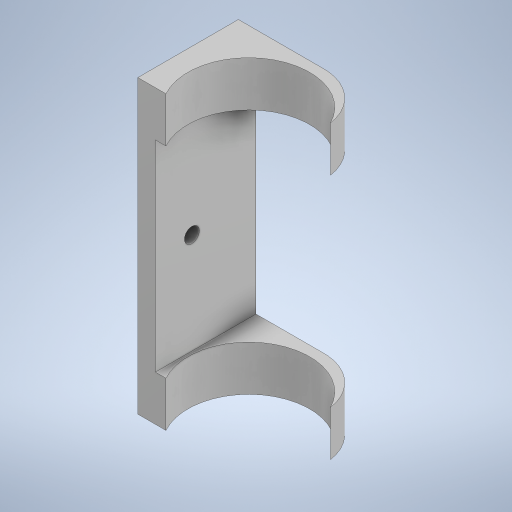
# Autodesk Inventor part: Speed Champ
Saved by Autodesk Inventor 2024 (Build 280153000, 153)
## iProperties
Created: 2023-08-06
Part Number: Speed Champ
Material: Generic
Document SubType Name: Modeling
Designer: AdminForWorker
Density: 1 g/cm^3
Appearance: Default
Title: Speed Champ v1
Author: AdminForWorker
Autodesk Inventor part; units mm, degrees
ref_plane "YZ Plane" through (0, 0, 0) normal (1, 0, 0) x (0, 1, 0)
ref_plane "Work Plane1" through (-14.5, -35, 0) normal (0, -1, 0) x (1, 0, 0)
sketch "Sketch2" plane through (-14.5, -35, 0) normal (0, -1, 0) x (1, 0, 0)
  line L0 (4.3469, 0) -> (4.3469, 20)
  line L1 (7.596, 20) -> (7.4184, 20) projected
  line L2 (4.3469, 20) -> (7.596, 20)
  arc A0 (7.596, 20) -> (29, 8.6937) centre (18.17, 14.1045) ccw
  line L3 (4.3469, 0) -> (18.3998, 0)
  arc A1 (18.3998, 0) -> (29, 8.6937) centre (18.9461, 10.1431) ccw
  point P0 (14.5, 0)
  point P1 (5, 0)
  point P2 (18.2531, 1.9984)
  constraints: 6 end point, 5 point on circle, 2 centre point, 1 horizontal, 1 perpendicular
extrude "Extrusion1" add sketch "Sketch2" against normal blind 15
ref_plane "Work Plane4" through (-14.5, -35, 0) normal (-1, 0, 0) x (0, 0, 1)
sketch "Sketch3" plane through (-14.5, -35, 0) normal (-1, 0, 0) x (0, 0, 1)
  line L0 (20, 0) -> (20, 70) projected
  line L1 (0, 0) -> (0, 21) projected
  line L2 (20, 70) -> (0, 70)
  line L3 (0, 70) -> (0, 0)
  line L4 (0, 0) -> (20, 0)
  line L5 (20, 0) -> (20, 70)
  point P0 (0, 35)
  constraints: 8 end point, 2 parallel, 1 horizontal, 1 perpendicular
extrude "Extrusion2" add sketch "Sketch3" against normal blind 5.5
mirror "Mirror3" about plane through (0, 0, 0) normal (0, 1, 0) of "Extrusion1"
sketch "Sketch4" plane through (-9, -35, 0) normal (1, 0, 0) x (0, 0, -1)
  line L0 (-20, 15) -> (-1.9981, 15) projected
  line L1 (-12.7438, 15) -> (-12.7438, 55)
  line L2 (0, 55) -> (-20, 55) projected
  line L3 (-12.7438, 35) -> (-17.7089, 35)
  circle A0 centre (-12.7438, 35) radius 1.5
  point P0 (0, 35)
  point P1 (-8.6937, 15)
  dimension "d4" = 3
  constraints: 4 end point, 2 point on line, 1 centre point, 1 coincident, 1 horizontal, 1 midpoint, 1 vertical
  measures "d4" diameter of A0
extrude "Extrusion3" cut sketch "Sketch4" against normal blind 10.375
sketch "Sketch5" plane through (-14.5, -35, 0) normal (-1, 0, 0) x (0, 0, 1)
  line L0 (20, 70) -> (0, 70) projected
  line L1 (0, 0) -> (20, 0) projected
  line L2 (20, 70) -> (0, 70)
  line L3 (0, 70) -> (0, 0)
  line L4 (0, 0) -> (20, 0)
  line L5 (20, 0) -> (20, 70)
  point P0 (0, 35)
  constraints: 8 end point, 2 parallel, 1 horizontal, 1 perpendicular
extrude "Extrusion4" cut sketch "Sketch5" against normal blind 2
sketch "Sketch7" plane through (-14.5, -35, 0) normal (0, -1, 0) x (1, 0, 0)
  line L0 (7.596, 20) -> (2, 20) projected
  line L1 (2, 20) -> (2, 0) projected
  line L2 (2, 20) -> (2, 0)
  arc A0 (18.3998, 0) -> (29, 8.6937) centre (18.9461, 10.1431) ccw projected
  line L3 (5.5, 20) -> (7.596, 20) projected
  arc A1 (7.596, 20) -> (29, 8.6937) centre (18.17, 14.1045) ccw
  arc A2 (7.596, 20) -> (29, 8.6937) centre (18.17, 14.1045) ccw projected
  arc A3 (19.4924, 0) -> (29, 8.6937) centre (18.9461, 10.1431) ccw
  line L4 (2, 20) -> (7.596, 20)
  line L5 (2, 0) -> (18.3998, 0) projected
  line L6 (2, 0) -> (18.3998, 0)
  point P0 (14.5, 0)
  constraints: 6 end point, 5 point on circle, 2 centre point, 2 concentric, 1 collinear, 1 vertical
extrude "Extrusion5" cut sketch "Sketch7" against normal blind 6
sketch "Sketch8" plane through (-12.5, 35, 0) normal (0, 1, 0) x (1, 0, 0)
  line L0 (3.5, -20) -> (5.596, -20) projected
  line L1 (0, 0) -> (0, -20) projected
  line L2 (5.596, -20) -> (0, -20)
  line L3 (0, -20) -> (0, 0)
  arc A0 (27, -8.6937) -> (16.3998, 0) centre (16.9461, -10.1431) ccw projected
  line L4 (0, 0) -> (16.3998, 0)
  arc A1 (27, -8.6937) -> (5.596, -20) centre (16.17, -14.1045) ccw projected
  arc A2 (27, -8.6937) -> (5.596, -20) centre (16.17, -14.1045) ccw
  arc A3 (27, -8.6937) -> (16.3998, 0) centre (16.9461, -10.1431) ccw
  point P0 (12.5, 0)
  constraints: 6 end point, 4 point on circle, 2 centre point, 2 perpendicular, 1 collinear, 1 concentric
extrude "Extrusion6" cut sketch "Sketch8" against normal blind 6
body "Solid1"
body "Solid3"
